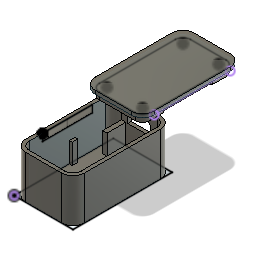
esp12_box v5 (Autodesk Fusion 360 design; units mm, degrees)
Autodesk Fusion 360 part; units mm, degrees
sketch "Base" plane through (0, 0, 0) normal (0, 1, 0) x (1, 0, 0) in component "Case"
  line L0 (0, 0) -> (20.4, 0)
  line L1 (20.4, 0) -> (20.4, 34.4)
  line L2 (20.4, 34.4) -> (0, 34.4)
  line L3 (0, 34.4) -> (0, 0)
  dimension "d6" = 20.4
  dimension "d7" = 34.4
  constraint horizontal L0
  constraint vertical L1
  constraint horizontal L2
  constraint vertical L3
  constraint coincident L0.start L3.end
  measures "d6" distance of L0.start L0.end
  measures "d7" distance of L0.start L2.end
extrude "Extrude1" add sketch "Base" along normal blind 15 makes body 1 in component "Case"
fillet "Fillet1" radius 4 4 edges at (20.4, 7.5, 0) (0, 7.5, 0) (20.4, 7.5, -34.4) (0, 7.5, -34.4) on bodies 1 in component "Case"
shell "Shell1" thickness 1.2 removed faces 1 at (6.8, 15, -21.6) on bodies 1 in component "Case"
sketch "Knob" plane through (1.2, 0, 0) normal (1, 0, 0) x (0, 0, -1) in component "Case"
  line L0 (30.4, 1.2) -> (30.4, 15)
  line L1 (30.4, 15) -> (4, 15)
  line L2 (4, 15) -> (4, 1.2)
  line L3 (4, 1.2) -> (30.4, 1.2)
  line L4 (8.6, 15) -> (25.8, 15)
  line L5 (25.8, 15) -> (25.8, 12.6)
  line L6 (25.8, 12.6) -> (8.6, 12.6)
  line L7 (8.6, 12.6) -> (8.6, 15)
  line L8 (17.2, 15) -> (17.2, 12.6) construction
  dimension "d12" = 17.2
  dimension "d13" = 2.4
  constraint horizontal L4
  constraint vertical L5
  constraint horizontal L6
  constraint vertical L7
  constraint coincident L1 L4.start
  constraint midpoint L1 L8.start
  constraint midpoint L6 L8.end
  constraint vertical L8
  measures "d12" distance of L5.end L6.end
  measures "d13" distance of L4.end L5.end
extrude "Extrude2" add sketch "Knob" along normal blind 6 draft -45 contours L1 L4 L5 L6 L7 bodies 1 in component "Case"
ref_plane "WorkPlane2" through (10.2, 7.5, -17.2) normal (-1, 0, 0) x (0, 0, 1) in component "Case"
mirror "Mirror1" about plane through (10.2, 7.5, -17.2) normal (-1, 0, 0) of "Extrude2" in component "Case"
sketch "Top" plane through (0, 15, 0) normal (0, 1, 0) x (-1, 0, 0) in component "Top Cover"
  line L0 (-20.4, -4) -> (-20.4, -30.4)
  arc A0 (-20.4, -30.4) -> (-16.4, -34.4) centre (-16.4, -30.4) ccw
  line L1 (-16.4, -34.4) -> (-4, -34.4)
  arc A1 (-4, -34.4) -> (0, -30.4) centre (-4, -30.4) ccw
  line L2 (0, -30.4) -> (0, -4)
  arc A2 (0, -4) -> (-4, 0) centre (-4, -4) ccw
  line L3 (-4, 0) -> (-16.4, 0)
  arc A3 (-16.4, 0) -> (-20.4, -4) centre (-16.4, -4) ccw
  line L4 (-19.2, -8.6) -> (-19.2, -4)
  arc A4 (-16.4, -1.2) -> (-19.2, -4) centre (-16.4, -4) ccw
  line L5 (-16.4, -1.2) -> (-4, -1.2)
  arc A5 (-1.2, -4) -> (-4, -1.2) centre (-4, -4) ccw
  line L6 (-1.2, -4) -> (-1.2, -8.6)
  line L7 (-1.2, -8.6) -> (-1.2, -25.8)
  line L8 (-1.2, -25.8) -> (-1.2, -30.4)
  arc A6 (-4, -33.2) -> (-1.2, -30.4) centre (-4, -30.4) ccw
  line L9 (-4, -33.2) -> (-16.4, -33.2)
  arc A7 (-19.2, -30.4) -> (-16.4, -33.2) centre (-16.4, -30.4) ccw
  line L10 (-19.2, -30.4) -> (-19.2, -25.8)
  line L11 (-19.2, -25.8) -> (-19.2, -8.6)
extrude "Extrude1'" add sketch "Top" along normal blind 1.2 separate body contours L0 A0 L1 A1 L2 A2 L3 A3 | L4 A4 L5 A5 L6 L7 L8 A6 L9 A7 L10 L11 makes body 2 in component "Top Cover"
sketch "Lip" plane through (0, 15, 0) normal (0, -1, 0) x (1, 0, 0) in component "Top Cover"
  arc A0 (20.4, -4) -> (16.4, 0) centre (16.4, -4) ccw
  line L0 (16.4, 0) -> (4, 0)
  arc A1 (4, 0) -> (0, -4) centre (4, -4) ccw
  line L1 (0, -4) -> (0, -30.4)
  arc A2 (0, -30.4) -> (4, -34.4) centre (4, -30.4) ccw
  line L2 (4, -34.4) -> (16.4, -34.4)
  arc A3 (16.4, -34.4) -> (20.4, -30.4) centre (16.4, -30.4) ccw
  line L3 (20.4, -30.4) -> (20.4, -4)
  line L4 (19, -30.4) -> (19, -4)
  arc A4 (19, -4) -> (16.4, -1.4) centre (16.4, -4) ccw
  line L5 (16.4, -1.4) -> (4, -1.4)
  arc A5 (4, -1.4) -> (1.4, -4) centre (4, -4) ccw
  line L6 (1.4, -4) -> (1.4, -30.4)
  arc A6 (1.4, -30.4) -> (4, -33) centre (4, -30.4) ccw
  line L7 (4, -33) -> (16.4, -33)
  arc A7 (16.4, -33) -> (19, -30.4) centre (16.4, -30.4) ccw
  line L8 (20.4, -4) -> (20.4, -30.4)
  dimension "d19" = 1.4
  dimension "d31" = 1.4
  measures "d31" distance of L4 L8
extrude "Extrude2'" add sketch "Lip" along normal blind 2.4 contours L4 A4 L5 A5 L6 A6 L7 A7 bodies 2 in component "Top Cover"
extrude "Extrude3" cut sketch "Knob" along normal blind 2.4 draft -45 from surface at 0.2 contours L1 L4 L5 L6 L7 bodies 2 in component "Top Cover"
ref_plane "WorkPlane2" through (10.2, 0, 0) normal (1, 0, 0) x (0, 1, 0) in component "Top Cover"
mirror "Mirror1'" about plane through (10.2, 0, 0) normal (1, 0, 0) of "Extrude3" in component "Top Cover"
shell "Shell1'" thickness 1.2 removed faces 1 at (13.1333, 12.6, -20.0667) on bodies 2 in component "Top Cover"
chamfer "Chamfer1" distance 0.6 angle 45 2 edges at (1.4, 12.6, -17.2) (19, 12.6, -17.2) on bodies 2 in component "Top Cover"
sketch "Esquisse1" plane through (0, 0, -34.4) normal (0, 0, -1) x (-1, 0, 0)
  line L0 (-4, 0) -> (-4, 15)
  line L1 (-4, 15) -> (-16.4, 15)
  line L2 (-16.4, 15) -> (-16.4, 0)
  line L3 (-16.4, 0) -> (-4, 0)
  line L4 (-6.2, 12.2) -> (-14.2, 12.2)
  line L5 (-14.2, 12.2) -> (-14.2, 8.2)
  line L6 (-14.2, 8.2) -> (-6.2, 8.2)
  line L7 (-6.2, 8.2) -> (-6.2, 12.2)
  line L8 (-6.2, 12.2) -> (-14.2, 8.2) construction
  line L9 (-14.2, 12.2) -> (-6.2, 8.2) construction
  line L10 (0, 0) -> (0, 15)
  line L11 (-20.4, 0) -> (0, 0)
  point P0 (-10.2, 10.2)
  dimension "d36" = 8
  dimension "d37" = 4
  dimension "d38" = 10.2
  dimension "d43" = 10.2
  constraint horizontal L4
  constraint perpendicular L4 L5
  constraint parallel L4 L6
  constraint parallel L5 L7
  constraint coincident L8 P0
  constraint coincident L9 P0
  measures "d36" distance of L5.end L6.end
  measures "d37" distance of L4.end L5.end
  measures "d38" distance of P0 L10
  measures "d43" distance of P0 L11
extrude "Extrusion3" cut sketch "Esquisse1" against normal blind 2.2 contours L4 L5 L6 L7 bodies 1 in component "Case"
fillet "Congé3" radius 1.5 2 edges at (6.2, 12.2, -33.8) (14.2, 12.2, -33.8) on bodies 1 in component "Case"
sketch "Esquisse2" plane through (0, 1.2, 0) normal (0, 1, 0) x (-1, 0, 0)
  arc A0 (-4, -33.2) -> (-1.2, -30.4) centre (-4, -30.4) ccw
  line L0 (-1.2, -30.4) -> (-1.2, -4)
  arc A1 (-1.2, -4) -> (-4, -1.2) centre (-4, -4) ccw
  line L1 (-4, -1.2) -> (-16.4, -1.2)
  arc A2 (-16.4, -1.2) -> (-19.2, -4) centre (-16.4, -4) ccw
  line L2 (-19.2, -4) -> (-19.2, -30.4)
  arc A3 (-19.2, -30.4) -> (-16.4, -33.2) centre (-16.4, -30.4) ccw
  line L3 (-16.4, -33.2) -> (-4, -33.2)
  line L4 (-16.5014, -33.2) -> (-15.0014, -33.2)
  line L5 (-15.0014, -33.2) -> (-15.0014, -26.7)
  line L6 (-15.0014, -26.7) -> (-16.5014, -26.7)
  line L7 (-16.5014, -26.7) -> (-16.5014, -33.2)
  line L8 (-4, -33.2) -> (-5.5, -33.2)
  line L9 (-5.5, -33.2) -> (-5.5, -26.7)
  line L10 (-5.5, -26.7) -> (-4, -26.7)
  line L11 (-4, -26.7) -> (-4, -33.2)
  line L12 (-19.2, -19.9445) -> (-18.2, -19.9445)
  line L13 (-18.2, -19.9445) -> (-18.2, -17.9445)
  line L14 (-18.2, -17.9445) -> (-19.2, -17.9445)
  line L15 (-19.2, -17.9445) -> (-19.2, -19.9445)
  line L16 (-1.2, -19.9102) -> (-2.2, -19.9102)
  line L17 (-2.2, -19.9102) -> (-2.2, -17.9102)
  line L18 (-2.2, -17.9102) -> (-1.2, -17.9102)
  line L19 (-1.2, -17.9102) -> (-1.2, -19.9102)
  line L20 (-19.2, -8.0198) -> (-18.2, -8.0198)
  line L21 (-18.2, -8.0198) -> (-18.2, -6.0198)
  line L22 (-18.2, -6.0198) -> (-19.2, -6.0198)
  line L23 (-19.2, -6.0198) -> (-19.2, -8.0198)
  line L24 (-1.2, -7.9308) -> (-2.2, -7.9308)
  line L25 (-2.2, -7.9308) -> (-2.2, -5.9308)
  line L26 (-2.2, -5.9308) -> (-1.2, -5.9308)
  line L27 (-1.2, -5.9308) -> (-1.2, -7.9308)
  dimension "d44" = 1.5
  dimension "d45" = 6.5
  dimension "d46" = 1.5
  dimension "d47" = 6.5
  dimension "d65" = 1
  dimension "d66" = 2
  dimension "d67" = 1
  dimension "d68" = 2
  dimension "d69" = 1
  dimension "d70" = 2
  dimension "d71" = 1
  dimension "d72" = 2
  constraint horizontal L4
  constraint vertical L5
  constraint horizontal L6
  constraint vertical L7
  constraint coincident L3 L4.start
  constraint horizontal L8
  constraint vertical L9
  constraint horizontal L10
  constraint vertical L11
  constraint coincident A0.start L3.end
  constraint horizontal L12
  constraint vertical L13
  constraint horizontal L14
  constraint vertical L15
  constraint coincident L2 L12.start
  constraint horizontal L16
  constraint vertical L17
  constraint horizontal L18
  constraint vertical L19
  constraint coincident L0 L16.start
  constraint horizontal L20
  constraint vertical L21
  constraint horizontal L22
  constraint vertical L23
  constraint coincident L2 L20.start
  constraint horizontal L24
  constraint vertical L25
  constraint horizontal L26
  constraint vertical L27
  constraint coincident L0 L24.start
  measures "d44" distance of L4.start L4.end
  measures "d45" distance of L4.start L6.end
  measures "d46" distance of A0.start L8.end
  measures "d47" distance of A0.start L10.end
  measures "d65" distance of L12.start L12.end
  measures "d66" distance of L12.start L14.end
  measures "d67" distance of L16.start L16.end
  measures "d68" distance of L16.start L18.end
  measures "d69" distance of L20.start L20.end
  measures "d70" distance of L20.start L22.end
  measures "d71" distance of L24.start L24.end
  measures "d72" distance of L24.start L26.end
extrude "Extrusion4" add sketch "Esquisse2" along normal blind 7 contours L3 L8 L9 L10 L11 | L0 L16 L17 L18 L19 | A3 L3 L4 L5 L6 L7 | L0 L24 L25 L26 L27 | L2 L12 L13 L14 L15 | L2 L20 L21 L22 L23 bodies 1 in component "Case"
sketch "Esquisse3" plane through (0, 32.9595, 0) normal (0, 1, 0) x (-1, 0, 0)
  line L0 (-45.0409, -24.6464) -> (-45.0409, -51.0464)
  arc A0 (-45.0409, -51.0464) -> (-41.0409, -55.0464) centre (-41.0409, -51.0464) ccw
  line L1 (-41.0409, -55.0464) -> (-28.6409, -55.0464)
  arc A1 (-28.6409, -55.0464) -> (-24.6409, -51.0464) centre (-28.6409, -51.0464) ccw
  line L2 (-24.6409, -51.0464) -> (-24.6409, -24.6464)
  arc A2 (-24.6409, -24.6464) -> (-28.6409, -20.6464) centre (-28.6409, -24.6464) ccw
  line L3 (-28.6409, -20.6464) -> (-41.0409, -20.6464)
  arc A3 (-41.0409, -20.6464) -> (-45.0409, -24.6464) centre (-41.0409, -24.6464) ccw
  circle A4 centre (-33.6409, -38.6464) radius 1.8
  dimension "d50" = 3.6
  dimension "d51" = 18
  dimension "d52" = 9
  measures "d50" diameter of A4
  measures "d51" distance of L3 A4.centre
  measures "d52" distance of L2 A4.centre
extrude "Extrusion4'" [suppressed] in component "Top Cover"
fillet "Congé1" [suppressed] in component "Top Cover"
component "Enclosure" placed x (1, 0, 0) y (0, 1, 0) z (0, 0, 1) at (0, 0, 0)
component "Case" placed x (1, 0, 0) y (0, 1, 0) z (0, 0, 1) at (0, 0, 0) in component "Enclosure"
component "Top Cover" placed x (1, 0, 0) y (0, 1, 0) z (0, 0, 1) at (24.6409, 16.7595, -20.6464) in component "Enclosure"
equation "Width = Width_internal + ( 2 * shell )"
equation "length = Length_internal + ( 2 * shell )"
equation "heigth = 15 mm"
equation "shell = 1.2 mm"
equation "gap = 0.2 mm"
equation "d6 = length"
equation "d7 = Width"
equation "d8 = heigth"
equation "d11 = shell"
equation "d12 = Width / 2"
equation "d13 = shell * 2"
equation "d17 = shell"
equation "d19 = shell + gap"
equation "d20 = shell * 2"
equation "d23 = shell * 2"
equation "d26 = shell"
equation "d31 = shell + gap"
equation "d33 = length / 2"
equation "Width_internal = 32 mm"
equation "Length_internal = 18 mm"
equation "d38 = length / 2"
equation "d41 = -shell - 1 mm"
equation "d43 = 9 mm + shell"
equation "d53 = -shell - 0.2 mm"
